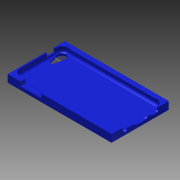
# Autodesk Inventor part: ipodcasev3
Saved by Autodesk Inventor 2014 SP1 (Build 180222100, 222)
## iProperties
Created: 2013-11-12
Part Number: ipodcasev3
Material: Generic
Document SubType Name: Modeling
Designer: jared.hale
Density: 1 g/cm^3
Appearance: Blue - Wall Paint - Glossy
Author: jared.hale
Autodesk Inventor part; units mm, degrees
ref_plane "YZ Plane" through (0, 0, 0) normal (1, 0, 0) x (0, 1, 0)
ref_plane "XZ Plane" through (0, 0, 0) normal (0, 1, 0) x (-1, 0, 0)
ref_plane "XY Plane" through (0, 0, 0) normal (0, 0, 1) x (1, 0, 0)
sketch "Sketch1" plane through (0, 0, 0) normal (0, 1, 0) x (-1, 0, 0)
  line L0 (-133.35, 69.85) -> (0, 69.85)
  line L1 (0, 69.85) -> (0, 0)
  line L2 (0, 0) -> (-133.35, 0)
  line L3 (-133.35, 0) -> (-133.35, 69.85)
  dimension "d0" = 133.35
  dimension "d2" = 69.85
  constraints: 8 end point, 2 parallel, 1 horizontal, 1 perpendicular
  measures "d0" distance between parallel lines of L1 L3
  measures "d2" distance between parallel lines of L2 L0
extrude "Extrusion1" add sketch "Sketch1" along normal blind 25.4
sketch "Sketch2" plane through (0, 25.4, 0) normal (0, 1, 0) x (1, 0, 0)
  line L0 (0, 0) -> (0, -69.85) projected
  line L1 (133.35, 0) -> (0, 0) projected
  line L2 (12.7, -5.08) -> (121.285, -5.08)
  line L3 (128.905, -12.7) -> (128.905, -56.388)
  line L4 (121.285, -64.008) -> (12.7, -64.008)
  line L5 (5.08, -56.388) -> (5.08, -12.7)
  arc A0 (12.7, -5.08) -> (5.08, -12.7) centre (12.7, -12.7) ccw
  arc A1 (5.08, -56.388) -> (12.7, -64.008) centre (12.7, -56.388) ccw
  arc A2 (121.285, -64.008) -> (128.905, -56.388) centre (121.285, -56.388) ccw
  arc A3 (128.905, -12.7) -> (121.285, -5.08) centre (121.285, -12.7) ccw
  dimension "d5" = 58.928
  dimension "d7" = 123.825
  dimension "d8" = 5.08
  dimension "d9" = 5.08
  dimension "d10" = 7.62
  constraints: 8 end point, 8 point on circle, 8 tangent, 4 centre point, 3 equal radius, 2 parallel, 1 horizontal, 1 perpendicular
  measures "d5" distance between parallel lines of L4 L2
  measures "d7" distance between parallel lines of L3 L5
  measures "d8" distance between parallel lines of L2 L1
  measures "d9" distance between parallel lines of L0 L5
  measures "d10" radius of A0
extrude "Extrusion2" cut sketch "Sketch2" against normal blind 6.4008
fillet "Fillet1" radius 3.175 8 edges at (126.6732, 18.9992, 7.3118) (128.905, 18.9992, 34.544) (126.6732, 18.9992, 61.7762) (66.9925, 18.9992, 64.008) (7.3118, 18.9992, 61.7762) (5.08, 18.9992, 34.544) (7.3118, 18.9992, 7.3118) (66.9925, 18.9992, 5.08)
sketch "Sketch3" plane through (5.08, 25.4, 56.388) normal (1, 0, 0) x (0, 0, -1)
  line L0 (43.688, 0) -> (43.688, -3.2258) projected
  line L1 (32.893, 1.737) -> (42.672, 1.737)
  line L2 (42.672, 1.737) -> (42.672, -4.445)
  line L3 (42.672, -4.445) -> (32.893, -4.445)
  line L4 (32.893, -4.445) -> (32.893, 1.737)
  point P0 (56.388, -25.4)
  dimension "d14" = 1.016
  dimension "d15" = 9.779
  constraints: 8 end point, 2 parallel, 1 horizontal, 1 perpendicular
  measures "d14" distance between parallel lines of L2 L0
  measures "d15" distance between parallel lines of L4 L2
extrude "Extrusion3" cut sketch "Sketch3" along normal mid plane 50.8
sketch "Sketch4" plane through (121.285, 25.4, 64.008) normal (0, 0, -1) x (-1, 0, 0)
  line L0 (0, 0) -> (108.585, 0) projected
  line L1 (76.581, -4.953) -> (101.981, -4.953)
  line L2 (101.981, -4.953) -> (101.981, 0.8392)
  line L3 (101.981, 0.8392) -> (76.581, 0.8392)
  line L4 (76.581, 0.8392) -> (76.581, -4.953)
  point P0 (108.585, -3.2258)
  point P1 (121.285, -25.4)
  point P2 (116.205, -3.2258)
  dimension "d37" = 7.62
  dimension "d38" = 14.224
  dimension "d39" = 25.4
  dimension "d40" = 5.7912
  dimension "d41" = 3.2258
  constraints: 8 end point, 2 parallel, 1 horizontal, 1 perpendicular
  measures "d37" distance of point (108.585, -3.226) point (116.205, -3.226)
  measures "d38" distance from line of point (116.205, -3.226) L2
  measures "d39" distance between parallel lines of L4 L2
  measures "d41" distance from line of point (116.205, -3.226) L0
sketch "Sketch5" plane through (128.905, 25.4, 12.7) normal (-1, 0, 0) x (0, 0, 1)
  line L0 (43.688, -3.2258) -> (0, -3.2258) projected
  line L1 (0, 0) -> (43.688, 0) projected
  ellipse E0 centre (21.7805, -3.175) end of major axis (30.6705, -3.175) minor radius 2.54
  point P0 (-12.7, -25.4)
  dimension "d21" = 8.89
  dimension "d23" = 2.54
  dimension "d26" = 3.175
  constraints: 1 horizontal, 2 other
  measures "d26" distance from line of point (21.78, -3.175) L1
extrude "Extrusion4" cut sketch "Sketch5" along normal mid plane 50.8
sketch "Sketch6" plane through (128.905, 25.4, 12.7) normal (-1, 0, 0) x (0, 0, 1)
  ellipse E0 centre (21.7805, -3.175) end of major axis (12.8905, -3.175) minor radius 2.54 (30.6687, -3.2258) -> (12.8923, -3.2258) ccw projected
  line L0 (12.8923, -3.2258) -> (0, -3.2258) projected
  circle A0 centre (40.7035, -3.175) radius 2.9845
  ellipse E1 centre (5.2705, -3.175) end of major axis (10.541, -3.175) minor radius 1.905
  line L1 (0, 0) -> (0, -3.2258) projected
  line L2 (43.688, 0) -> (43.688, -3.2258) projected
  point P0 (-12.7, -25.4)
  dimension "d36" = 1.905
  dimension "d31" = 18.923
  dimension "d34" = 16.51
  constraints: 1 centre point, 1 horizontal, 1 tangent, 1 vertical, 3 other
  measures "d31" distance of point (21.78, -3.175) A0.centre
  measures "d34" distance of point (5.27, -3.175) point (21.78, -3.175)
extrude "Extrusion5" cut sketch "Sketch6" along normal mid plane 10.16
extrude "Extrusion6" cut sketch "Sketch4" along normal mid plane 50.8
sketch "Sketch7" plane through (0, 18.9992, 0) normal (0, 1, 0) x (1, 0, 0)
  line L0 (12.7, -8.255) -> (121.285, -8.255) projected
  line L1 (8.255, -56.388) -> (8.255, -12.7) projected
  arc A0 (16.7866, -12.9365) -> (7.3434, -12.9365) centre (12.065, -11.938) ccw
  arc A1 (9.58, -23.5125) -> (14.55, -23.5125) centre (12.065, -22.987) ccw
  line L2 (7.3434, -12.9365) -> (9.58, -23.5125)
  line L3 (16.7866, -12.9365) -> (14.55, -23.5125)
  point P0 (0, 0)
  point P1 (5.08, -5.08)
  dimension "d46" = 11.049
  dimension "d48" = 0
  dimension "d49" = 9.652
  dimension "d50" = 5.08
  dimension "d51" = 3.175
  dimension "d52" = 3.175
  dimension "d53" = 6.858
  dimension "d54" = 6.985
  constraints: 4 end point, 4 point on circle, 4 tangent, 2 centre point
  measures "d46" distance of A1.centre A0.centre
  measures "d48" horizontal distance of A0.centre A1.centre
  measures "d49" diameter of A0
  measures "d50" diameter of A1
  measures "d51" distance from line of point (5.08, -5.08) L0
  measures "d52" distance from line of point (5.08, -5.08) L1
  measures "d53" vertical distance of A0.centre point (5.08, -5.08)
  measures "d54" horizontal distance of A0.centre point (5.08, -5.08)
extrude "Extrusion7" cut sketch "Sketch7" along normal mid plane 50.8
ref_plane "Work Plane1" through (0, 0, 34.925) normal (0, 0, 1) x (1, 0, 0)
sketch "Sketch10" plane through (0, 0, 34.925) normal (0, 0, 1) x (1, 0, 0)
  line L0 (15.1836, 18.9992) -> (121.285, 18.9992) projected
  line L1 (5.08, 24.13) -> (5.7032, 25.2095) projected
  line L2 (128.905, 24.13) -> (128.2818, 25.2095) projected
  line L3 (3.556, 25.8521) -> (3.556, 17.4752)
  line L4 (3.556, 17.4752) -> (130.429, 17.4752)
  line L5 (130.429, 17.4752) -> (130.429, 25.8521)
  line L6 (3.556, 25.8521) -> (-3.1756, 25.6598)
  line L7 (-3.1756, 25.6598) -> (-4.2851, -9.2303)
  line L8 (-4.2851, -9.2303) -> (140.2506, -12.8123)
  line L9 (140.2506, -12.8123) -> (141.3589, 31.9078)
  line L10 (141.3589, 31.9078) -> (130.429, 25.8521)
  point P0 (0, 0)
  dimension "d62" = 1.524
  dimension "d63" = 1.524
  dimension "d65" = 1.524
  constraints: 16 end point, 1 parallel, 1 perpendicular
  measures "d62" distance from line of L3 L1.start
  measures "d63" distance from line of L5 L2.start
  measures "d65" distance between parallel lines of L4 L0
extrude "Extrusion8" cut sketch "Sketch10" along normal mid plane 101.6
ref_plane "Work Plane2" through (66.9925, 22.1742, 43.3687) normal (-1, 0, 0) x (0, 0, 1)
chamfer "Chamfer3" distance 0.762 angle 45 4 edges at (12.065, 17.4752, 7.112) (15.6683, 17.4752, 18.2245) (12.065, 17.4752, 25.527) (8.4617, 17.4752, 18.2245)
ref_plane "Work Plane4" through (67.7545, 25.4, 56.388) normal (1, 0, 0) x (0, 0, -1)
sketch "Sketch20" plane through (67.7545, 25.4, 56.388) normal (1, 0, 0) x (0, 0, -1)
  line L0 (51.5623, 0) -> (51.5623, -7.9248) projected
  line L1 (51.308, 0) -> (51.308, -3.2258) projected
  line L2 (42.672, 0) -> (51.5623, 0) projected
  line L3 (51.308, -0.635) -> (50.673, 0)
  line L4 (50.673, 0) -> (51.308, 0)
  line L5 (51.308, 0) -> (51.308, -0.635)
  point P0 (56.388, -25.4)
  point P1 (51.5623, -4.5974)
  point P2 (44.3991, 0)
  point P3 (44.2622, 0)
  point P4 (42.4183, 0)
  dimension "d146" = 45
  dimension "d147" = 0.635
  constraints: 6 end point, 2 point on line, 1 collinear, 1 perpendicular
  measures "d146" angle of L3 L5
  measures "d147" distance from line of L1 L3.end
extrude "Extrusion16" add sketch "Sketch20" against normal up to surface round surface about axis through (12.7, 25.4, 12.7) along (0, -1, 0) radius 7.62 far side no
sketch "Sketch21" plane through (67.7545, 25.4, 56.388) normal (1, 0, 0) x (0, 0, -1)
  line L0 (51.308, 0) -> (50.673, 0) projected
  line L1 (50.673, 0) -> (51.308, -0.635) projected
  line L2 (50.673, 0) -> (51.308, -0.635)
  line L3 (50.673, 0) -> (51.308, 0)
  line L4 (51.308, 0) -> (51.308, -0.635)
  point P0 (56.388, -25.4)
  constraints: 6 end point, 1 collinear, 1 perpendicular, 1 point on line
extrude "Extrusion17" add sketch "Sketch21" along normal up to surface round surface about axis through (121.285, 25.4, 12.7) along (0, -1, 0) radius 7.62 far side no
ref_plane "Work Plane5" through (12.7, 22.1742, 34.544) normal (0, 0, 1) x (1, 0, 0)
mirror "Mirror1" about plane through (12.7, 22.1742, 34.544) normal (0, 0, 1) of "Extrusion16", "Extrusion17"
sketch "Sketch23" plane through (128.905, 25.4, 12.7) normal (-1, 0, 0) x (0, 0, 1)
  arc A0 (43.6876, -3.2258) -> (37.7194, -3.2258) centre (40.7035, -3.175) ccw projected
  line L0 (43.688, -3.2258) -> (43.6876, -3.2258) projected
  line L1 (43.688, 0) -> (43.688, -3.2258) projected
  line L2 (0, 0) -> (43.688, 0) projected
  line L3 (0, 0) -> (0, -3.2258) projected
  ellipse E0 centre (5.2705, -3.175) end of major axis (0, -3.175) minor radius 1.905 (10.5391, -3.2258) -> (0.0019, -3.2258) ccw projected
  line L4 (12.8923, -3.2258) -> (10.5391, -3.2258) projected
  ellipse E1 centre (21.7805, -3.175) end of major axis (12.8905, -3.175) minor radius 2.54 (30.6687, -3.2258) -> (12.8923, -3.2258) ccw projected
  line L5 (37.7194, -3.2258) -> (30.6687, -3.2258) projected
  point P0 (0, -2.7642)
  point P1 (-12.7, -25.4)
  constraints: 2 other
extrude "Extrusion18" [suppressed]
sketch "Sketch24" plane through (128.905, 25.4, 12.7) normal (-1, 0, 0) x (0, 0, 1)
  arc A0 (43.688, -3.175) -> (37.7194, -3.2258) centre (40.7035, -3.175) ccw projected
  line L0 (43.688, 0) -> (43.688, -3.175) projected
  line L1 (0, 0) -> (43.688, 0) projected
  line L2 (0, 0) -> (0, -3.175) projected
  ellipse E0 centre (5.2705, -3.175) end of major axis (0, -3.175) minor radius 1.905 (10.5391, -3.2258) -> (0, -3.175) ccw projected
  line L3 (12.8923, -3.2258) -> (10.5391, -3.2258) projected
  ellipse E1 centre (21.7805, -3.175) end of major axis (12.8905, -3.175) minor radius 2.54 (30.6687, -3.2258) -> (12.8923, -3.2258) ccw projected
  line L4 (37.7194, -3.2258) -> (30.6687, -3.2258) projected
  point P0 (-12.7, -25.4)
  constraints: 2 other
extrude "Extrusion19" cut sketch "Sketch24" against normal through all
sketch "Sketch25" plane through (19.304, 25.4, 64.008) normal (0, 0, 1) x (1, 0, 0)
  line L0 (25.4, -0.635) -> (25.4, 0) projected
  line L1 (25.4, 0) -> (0, 0) projected
  line L2 (0, 0) -> (25.4, 0)
  line L3 (25.4, 0) -> (25.4, -0.635)
  line L4 (25.4, -0.635) -> (0, -0.635)
  line L5 (0, -0.635) -> (0, 0)
  point P0 (-19.304, -25.4)
  constraints: 8 end point, 2 parallel, 1 horizontal, 1 perpendicular
extrude "Extrusion20" cut sketch "Sketch25" against normal blind 25.4
ref_plane "Work Plane6" through (12.7, 17.4752, 4.8257) normal (0, -1, 0) x (1, 0, 0)
sketch "Sketch29" plane through (3.556, 17.4752, 0) normal (0, -1, 0) x (1, 0, 0)
  line L0 (126.873, 0) -> (0, 0) projected
  line L1 (126.873, 0) -> (126.873, 69.85) projected
  line L2 (0, 69.85) -> (126.873, 69.85) projected
  line L3 (0, 0) -> (0, 69.85) projected
  arc A0 (3.0419, 13.0941) -> (13.9761, 13.0941) centre (8.509, 11.938) ccw projected
  line L4 (5.2784, 23.6702) -> (3.0419, 13.0941) projected
  arc A1 (11.7396, 23.6702) -> (5.2784, 23.6702) centre (8.509, 22.987) ccw projected
  line L5 (13.9761, 13.0941) -> (11.7396, 23.6702) projected
  point P0 (-3.556, 0)
extrude "Extrusion21" add sketch "Sketch29" along normal blind 1.27
body "Solid1"
